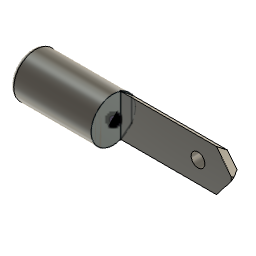
Interior Angle Connector v1 (Autodesk Fusion 360 design; units mm, degrees)
Autodesk Fusion 360 part; units mm, degrees
sketch "Sketch1" plane through (0, 0, 0) normal (1, 0, 0) x (0, 1, 0)
  circle A0 centre (0, 0) radius 11.303
  circle A1 centre (0, 0) radius 15.24
  line L0 (7.62, 13.1982) -> (7.62, -13.1982)
  line L1 (7.62, 13.1982) -> (15.24, 13.1982)
  line L2 (7.62, -13.1982) -> (15.24, -13.1982)
  line L3 (15.24, 13.1982) -> (15.24, -13.1982)
  dimension "d1" = 22.606
  dimension "d2" = 30.48
  dimension "d3" = 7.62
  dimension "d4" = 7.62
  dimension "d5" = 7.62
  constraint coincident A0.centre A1.centre
  constraint concentric A0 A1
  constraint coincident A1 L0.start
  constraint coincident A1 L0.end
  constraint vertical L0
  constraint perpendicular L0 L1
  constraint perpendicular L0 L2
  measures "d1" diameter of A0
  measures "d2" diameter of A1
  measures "d3" distance of A0.centre L0
  measures "d4" distance of L0.start L1.end
  measures "d5" distance of L0.end L2.end
extrude "Extrude1" add sketch "Sketch1" against normal blind 50.8 contours A0 A1 L0 | A0 A1 L0
fillet "Fillet1" radius 2.54 1 edges at (-50.8, -14.2087, 5.511)
extrude "Extrude2" add sketch "Sketch1" along normal blind 5.08 contours A0 L0 | A0 A1 L0 | A0 L0 | A0 A1 L0
sketch "Sketch2" plane through (5.08, 0, 0) normal (1, 0, 0) x (0, 1, 0)
  circle A0 centre (0, 0) radius 15.24
  circle A1 centre (0, 0) radius 15.24 construction
  line L0 (12.7, -8.4242) -> (12.7, 8.4242)
  line L1 (5.08, 13.97) -> (5.08, -14.3684)
  line L2 (5.08, 13.97) -> (5.08, 14.3684)
  line L3 (5.08, 14.3684) -> (12.7, 8.4242)
  line L4 (12.7, -8.4242) -> (5.08, -14.3684)
  dimension "d12" = 30.48
  dimension "d22" = 7.62
  dimension "d23" = 12.7
  constraint coincident A0.centre A1.centre
  constraint coincident A1 L0.start
  constraint coincident A1 L0.end
  constraint vertical L0
  constraint coincident A1 L1.end
  constraint vertical L1
  constraint coincident A1 L2.end
  constraint parallel L1 L2
  measures "d12" diameter of A1
  measures "d22" distance of L0 L1
  measures "d23" distance of A0.centre L0
extrude "Extrude3" add sketch "Sketch2" against normal blind 2.54 contours L0 L1 L2 L3 L4
extrude "Extrude4" add sketch "Sketch2" along normal blind 76.2 contours L0 L1 L2 L3 L4
sketch "Sketch4" plane through (0, 5.08, 0) normal (0, -1, 0) x (1, 0, 0)
  line L0 (5.08, 14.3684) -> (5.08, -14.3684)
  line L1 (5.08, -14.3684) -> (81.28, -14.3684)
  line L2 (81.28, -14.3684) -> (81.28, 14.3684)
  line L3 (81.28, 14.3684) -> (5.08, 14.3684)
  line L4 (81.28, 14.3684) -> (5.08, 14.3684)
  line L5 (5.08, 14.3684) -> (5.08, -14.3684)
  line L6 (5.08, -14.3684) -> (81.28, -14.3684)
  line L7 (81.28, -14.3684) -> (81.28, 14.3684)
  line L8 (5.08, 0) -> (58.42, 0) construction
  circle A0 centre (58.42, 0) radius 4.7625
  line L9 (19.54, 14.3684) -> (19.54, 0) construction
  line L10 (24.8737, 0) -> (24.8737, -14.3684) construction
  line L11 (58.42, 0) -> (58.42, 14.3684) construction
  line L12 (58.42, 4.7625) -> (81.28, 4.7625) construction
  line L13 (81.28, 4.7625) -> (81.28, -4.7625) construction
  line L14 (81.28, -4.7625) -> (58.42, -4.7625) construction
  line L15 (58.42, -4.7625) -> (58.42, 4.7625) construction
  line L16 (58.42, 14.3684) -> (81.28, 4.7625)
  line L17 (58.42, -4.7625) -> (58.42, -14.3684) construction
  line L18 (58.42, -14.3684) -> (81.28, -4.7625)
  dimension "d24" = 53.34
  dimension "d25" = 9.525
  dimension "d28" = 22.86
  dimension "d29" = 9.525
  constraint horizontal L4
  constraint vertical L5
  constraint horizontal L6
  constraint vertical L7
  constraint coincident L0.end L1.start
  constraint coincident L2.end L3.start
  constraint coincident L5 L8.start
  constraint perpendicular L2 L8
  constraint coincident L8.end A0.centre
  constraint coincident L4 L9.start
  constraint coincident L8 L9.end
  constraint perpendicular L8 L9
  constraint coincident L8 L10.start
  constraint coincident L6 L10.end
  constraint perpendicular L6 L10
  constraint equal L9 L10
  constraint coincident L4 L11.end
  constraint perpendicular L4 L11
  constraint horizontal L12
  constraint vertical L13
  constraint horizontal L14
  constraint vertical L15
  constraint coincident A0 L12.start
  constraint coincident L11 L12.start
  constraint coincident L6 L17.end
  constraint perpendicular L6 L17
  measures "d24" distance of L8.start L8.end
  measures "d25" diameter of A0
  measures "d28" distance of L12.start L12.end
  measures "d29" distance of L12.start L14.end
extrude "Extrude6" cut sketch "Sketch4" against normal blind 7.62 contours A0
chamfer "Chamfer1" distance 10.16 angle 45 2 edges at (81.28, 8.89, 11.3963) (81.28, 8.89, -11.3963)
